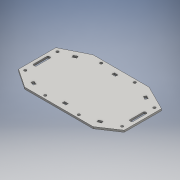
# Autodesk Inventor part: Support_Carte
Saved by Autodesk Inventor 2016 (Build 200138000, 138)
## iProperties
Created: 2016-09-30
Part Number: Support_Carte
Material: Générique
Document SubType Name: Modeling
Designer: LogOut
Density: 1 g/cm^3
Appearance: Par défaut
Author: LogOut
Autodesk Inventor part; units mm, degrees
ref_plane "YZ Plane" through (0, 0, 0) normal (1, 0, 0) x (0, 1, 0)
ref_plane "XZ Plane" through (0, 0, 0) normal (0, 1, 0) x (-1, 0, 0)
ref_plane "XY Plane" through (0, 0, 0) normal (0, 0, 1) x (1, 0, 0)
sketch "Esquisse1" plane through (0, 0, 0) normal (0, 0, 1) x (1, 0, 0)
  line L0 (110, -100) -> (-110, -100)
  line L1 (-170, -60) -> (-170, 60)
  line L2 (170, 60) -> (170, -60)
  line L3 (170, -100) -> (-170, 100) construction
  line L4 (-170, -100) -> (170, 100) construction
  line L5 (-90, 100) -> (-170, 60)
  line L6 (90, 100) -> (170, 60)
  line L7 (-170, -60) -> (-110, -100)
  line L8 (110, -100) -> (170, -60)
  line L9 (-90, 100) -> (90, 100)
  point P0 (0, 0)
  point P1 (0, 0)
  dimension "d0" = 340
  dimension "d1" = 80
  dimension "d2" = 40
  dimension "d3" = 80
  dimension "d4" = 40
  dimension "d5" = 40
  dimension "d6" = 60
  dimension "d7" = 60
  dimension "d8" = 40
  dimension "d17" = 100
  constraints: 20 end point, 6 point on line, 2 midpoint, 2 parallel, 1 horizontal, 1 perpendicular
  measures "d0" distance between parallel lines of L2 L1
  measures "d1" distance of L9.start L3.end
  measures "d2" distance of L1.end L3.end
  measures "d3" distance of L9.end L4.end
  measures "d4" distance of L2.start L4.end
  measures "d5" distance of L7.start L4.start
  measures "d6" distance of L7.end L4.start
  measures "d7" distance of L8.start L3.start
  measures "d8" distance of L8.end L3.start
  measures "d17" distance from line of point (0, 0) L0
extrude "Extrusion1" add sketch "Esquisse1" along normal blind 6
sketch "Esquisse2" plane through (0, 0, 6) normal (0, 0, 1) x (1, 0, 0)
  line L0 (-54, 90) -> (54, 90)
  line L1 (-156, 0) -> (156, 0)
  line L2 (-170, 60) -> (-170, -60)
  line L3 (170, -60) -> (170, 60)
  line L4 (-110, -100) -> (110, -100)
  line L5 (90, 100) -> (-69, 100)
  line L6 (-156, 0) -> (-156, 51.3475)
  line L7 (-156, 0) -> (-156, -52.5074)
  line L8 (156, 0) -> (156, 51.3475)
  line L9 (156, 0) -> (156, -52.5074)
  line L10 (170, 60) -> (90, 100) projected
  line L11 (110, -100) -> (170, -60) projected
  line L12 (-170, -60) -> (-110, -100) projected
  line L13 (-90, 100) -> (-170, 60) projected
  line L14 (90, 100) -> (-90, 100) projected
  point P0 (0, 0)
  point P1 (0, 0)
  point P2 (-54, -90)
  point P3 (54, -90)
  point P4 (0, 0)
  dimension "d21" = 14
  dimension "d22" = 14
  dimension "d23" = 10
  dimension "d24" = 108
  dimension "d25" = 54
  dimension "d29" = 108
  dimension "d30" = 10
  dimension "d31" = 10
  dimension "d32" = 56
  dimension "d34" = 56
  dimension "d42" = 14
  dimension "d43" = 14
  dimension "d44" = 14
  dimension "d45" = 14
  constraints: 20 end point, 4 vertical, 2 horizontal, 1 coincident, 1 collinear, 1 midpoint
  measures "d21" distance from line of L2 L1.start
  measures "d22" distance from line of L3 L8.start
  measures "d23" distance between parallel lines of L0 L5
  measures "d24" distance of L0.start L0.end
  measures "d25" horizontal distance of point (0, 0) L0.start
  measures "d29" distance of point (54, -90) point (-54, -90)
  measures "d30" distance from line of L4 point (54, -90)
  measures "d31" distance from line of L4 point (-54, -90)
  measures "d32" horizontal distance of L4.start point (-54, -90)
  measures "d34" horizontal distance of L4.end point (54, -90)
  measures "d42" distance from line of L10 L8.end
  measures "d43" distance from line of L11 L9.end
  measures "d44" distance from line of L12 L7.end
  measures "d45" distance from line of L13 L6.end
hole "Perçage1" at (-156, -52.5074, 6) at (-156, 51.3475, 6) at (-54, 90, 6) at (54, 90, 6) at (156, 51.3475, 6) at (156, -52.5074, 6) at (54, -90, 6) at (-54, -90, 6) direction (0, 0, -1) diameter 8 end through all
sketch "Esquisse3" plane through (0, 0, 6) normal (0, 0, 1) x (1, 0, 0)
  line L0 (-6, 84) -> (6, 84)
  line L1 (6, 84) -> (6, 76)
  line L2 (6, 76) -> (-6, 76)
  line L3 (-6, 76) -> (-6, 84)
  line L4 (-121.0377, 66.5926) -> (-110.3046, 71.9592)
  line L5 (-110.3046, 71.9592) -> (-106.7269, 64.8037)
  line L6 (-106.7269, 64.8037) -> (-117.46, 59.4372)
  line L7 (-117.46, 59.4372) -> (-121.0377, 66.5926)
  line L8 (-113.9841, -76.4747) -> (-102.7209, -80.6148)
  line L9 (-102.7209, -80.6148) -> (-99.9608, -73.106)
  line L10 (-99.9608, -73.106) -> (-111.2241, -68.9659)
  line L11 (-111.2241, -68.9659) -> (-113.9841, -76.4747)
  line L12 (-90, 100) -> (-170, 60) projected
  circle A0 centre (-156, 51.3475) radius 4 projected
  circle A1 centre (-156, -52.5074) radius 4 projected
  circle A2 centre (-54, -90) radius 4 projected
  line L13 (-156, -52.5074) -> (-54, -90)
  line L14 (0, 0) -> (0, -39.4059)
  line L15 (0, 0) -> (52.1624, 0)
  line L16 (121.0377, 66.5926) -> (110.3046, 71.9592)
  line L17 (110.3046, 71.9592) -> (106.7269, 64.8037)
  line L18 (106.7269, 64.8037) -> (117.46, 59.4372)
  line L19 (117.46, 59.4372) -> (121.0377, 66.5926)
  line L20 (113.9841, -76.4747) -> (102.7209, -80.6148)
  line L21 (102.7209, -80.6148) -> (99.9608, -73.106)
  line L22 (99.9608, -73.106) -> (111.2241, -68.9659)
  line L23 (111.2241, -68.9659) -> (113.9841, -76.4747)
  line L24 (156, -52.5074) -> (54, -90)
  line L25 (90, 100) -> (-90, 100) projected
  line L26 (-6, -84) -> (6, -84)
  line L27 (6, -84) -> (6, -76)
  line L28 (6, -76) -> (-6, -76)
  line L29 (-6, -76) -> (-6, -84)
  dimension "d46" = 16
  dimension "d47" = 24
  dimension "d48" = 12
  dimension "d49" = 38.089
  dimension "d52" = 8
  dimension "d53" = 12
  dimension "d54" = 47.705
  dimension "d55" = 12
  dimension "d56" = 8
  dimension "d57" = 6
  dimension "d58" = 16
  constraints: 56 end point, 14 symmetric about line, 7 parallel, 3 perpendicular, 2 collinear, 2 horizontal, 1 vertical
  measures "d46" distance between parallel lines of L12 L4
  measures "d47" distance between parallel lines of L12 L6
  measures "d48" distance between parallel lines of L7 L5
  measures "d49" distance from line of A0.centre L7
  measures "d52" distance between parallel lines of L8 L10
  measures "d53" distance between parallel lines of L11 L9
  measures "d54" distance from line of L13.start L11
  measures "d55" distance between parallel lines of L1 L3
  measures "d56" distance between parallel lines of L2 L0
  measures "d57" distance between parallel lines of L14 L3
  measures "d58" distance between parallel lines of L25 L0
extrude "Extrusion2" cut sketch "Esquisse3" against normal blind 10 contours L0 L1 L2 L3 | L4 L5 L6 L7 | L11 L10 L9 L8 | L19 L18 L17 L16 | L20 L21 L22 L23 | L29 L28 L27 L26
sketch "Esquisse4" plane through (0, 0, 6) normal (0, 0, 1) x (1, 0, 0)
  line L0 (0, 0) -> (0, 42.3404)
  line L1 (-152, 25) -> (-158, 25)
  line L2 (-160, 23) -> (-160, -23)
  line L3 (-158, -25) -> (-152, -25)
  line L4 (-150, -23) -> (-150, 23)
  line L5 (-158, 25) -> (-160, 23)
  line L6 (-152, 25) -> (-150, 23)
  line L7 (-152, -25) -> (-150, -23)
  line L8 (-160, -23) -> (-158, -25)
  line L9 (152, 25) -> (158, 25)
  line L10 (160, 23) -> (160, -23)
  line L11 (158, -25) -> (152, -25)
  line L12 (150, -23) -> (150, 23)
  line L13 (158, 25) -> (160, 23)
  line L14 (152, 25) -> (150, 23)
  line L15 (152, -25) -> (150, -23)
  line L16 (160, -23) -> (158, -25)
  point P0 (-150, 25)
  point P1 (-160, -25)
  point P2 (-160, 25)
  point P3 (-150, -25)
  point P4 (150, 25)
  point P5 (160, -25)
  point P6 (160, 25)
  point P7 (150, -25)
  dimension "d59" = 10
  dimension "d60" = 150
  dimension "d61" = 50
  dimension "d62" = 25
  dimension "d63" = 2
  dimension "d64" = 2
  dimension "d65" = 2
  dimension "d66" = 2
  dimension "d67" = 2
  dimension "d68" = 2
  dimension "d69" = 2
  dimension "d70" = 2
  constraints: 34 end point, 16 point on line, 12 symmetric about line, 2 parallel, 1 horizontal, 1 perpendicular, 1 vertical
  measures "d59" distance between parallel lines of L4 L2
  measures "d60" distance between parallel lines of L4 L0
  measures "d61" distance between parallel lines of L1 L3
  measures "d62" distance from line of L0.start L1
  measures "d63" distance of L1.end point (-160, 25)
  measures "d64" distance of L2.start point (-160, 25)
  measures "d65" distance of L1.start point (-150, 25)
  measures "d66" distance of L4.end point (-150, 25)
  measures "d67" distance of L3.end point (-150, -25)
  measures "d68" distance of L4.start point (-150, -25)
  measures "d69" distance of L2.end point (-160, -25)
  measures "d70" distance of L3.start point (-160, -25)
extrude "Extrusion3" cut sketch "Esquisse4" against normal blind 10
equation "\"d64\" = d63"
equation "\"d65\" = d63"
equation "\"d66\" = d65"
equation "\"d67\" = d63"
equation "\"d68\" = d67"
equation "\"d69\" = d63"
equation "\"d70\" = d69"
